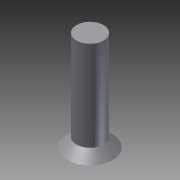
# Autodesk Inventor part: Tornillo tapa
Saved by Autodesk Inventor 2016 (Build 200138000, 138)
## iProperties
Created: 2013-07-10
Part Number: Tornillo tapa
Material: Generic
Document SubType Name: Modeling
Designer: Luis
Density: 1 g/cm^3
Appearance: Default
Author: Luis
Autodesk Inventor part; units mm, degrees
ref_plane "YZ Plane" through (0, 0, 0) normal (1, 0, 0) x (0, 1, 0)
ref_plane "XZ Plane" through (0, 0, 0) normal (0, 1, 0) x (-1, 0, 0)
ref_plane "XY Plane" through (0, 0, 0) normal (0, 0, 1) x (1, 0, 0)
sketch "Sketch1" plane through (0, 0, 0) normal (0, 0, 1) x (1, 0, 0)
  circle A0 centre (0, 0) radius 2.5
  circle A1 centre (0, 0) radius 1.5
  dimension "d0" = 5
  dimension "d1" = 3
  constraints: 2 centre point, 2 coincident
  measures "d0" diameter of A0
  measures "d1" diameter of A1
extrude "Extrusion1" add sketch "Sketch1" along normal blind 1
extrude "Extrusion2" add sketch "Sketch1" along normal blind 11 contours A1
chamfer "Chamfer1" distance 1 angle 45 1 edges at (-2.5, 0, 1)
sketch "Sketch2" plane through (0, 0, 0) normal (0, 0, -1) x (-1, 0, 0)
  circle A0 centre (0, 0) radius 2.5 projected
  line L0 (0.25, -1.5229) -> (-0.25, -1.5229)
  line L1 (-0.25, 1.4771) -> (0.25, 1.4771)
  line L2 (0.25, -1.4771) -> (-0.25, 1.4771) construction
  line L3 (1.5229, 0.25) -> (1.5229, -0.25)
  line L4 (-1.4771, -0.25) -> (-1.4771, 0.25)
  line L5 (1.4771, 0.25) -> (-1.4771, -0.25) construction
  line L6 (1.5229, -0.25) -> (0.25, -0.25)
  line L7 (-0.25, -0.25) -> (-1.4771, -0.25)
  line L8 (-1.4771, 0.25) -> (-0.25, 0.25)
  line L9 (0.25, 0.25) -> (1.5229, 0.25)
  line L10 (0.25, 1.4771) -> (0.25, 0.25)
  line L11 (0.25, -0.25) -> (0.25, -1.5229)
  line L12 (-0.25, -1.5229) -> (-0.25, -0.25)
  line L13 (-0.25, 0.25) -> (-0.25, 1.4771)
  point P0 (-1.3278, 0)
  dimension "d9" = 0.5
  dimension "d10" = 3
  dimension "d11" = 0.5
  dimension "d12" = 3
  constraints: 28 end point, 10 parallel, 4 perpendicular, 2 midpoint, 2 point on line, 1 coincident, 1 horizontal
  measures "d9" distance of L1.start L1.end
  measures "d10" distance of L0.end L1.start
  measures "d11" distance of L4.start L4.end
  measures "d12" distance of L3.end L4.start
extrude "Extrusion3" cut sketch "Sketch2" against normal blind 0.5 contours L0 L12 L7 L4 L8 L13 L1 L10 L9 L3 L6 L11
body "Solid1"
